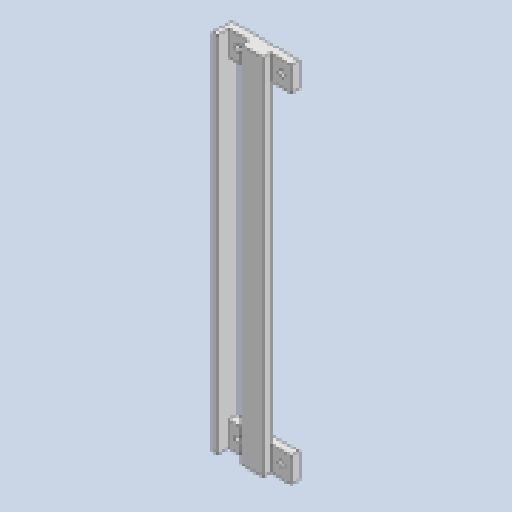
# Autodesk Inventor part: ex_shell_2_wid
Saved by Autodesk Inventor 2023 (Build 270158000, 158)
## iProperties
Created: 2022-10-02
Part Number: ex_shell_2_wid
Material: Generic
Document SubType Name: Modeling
Designer: Shuang Peng
Density: 1 g/cm^3
Appearance: Default
Author: Shuang Peng
Autodesk Inventor part; units mm, degrees
ref_plane "YZ Plane" through (0, 0, 0) normal (1, 0, 0) x (0, 1, 0)
ref_plane "XZ Plane" through (0, 0, 0) normal (0, 1, 0) x (-1, 0, 0)
ref_plane "XY Plane" through (0, 0, 0) normal (0, 0, 1) x (1, 0, 0)
sketch "Sketch1" plane through (0, 0, 0) normal (0, 0, 1) x (1, 0, 0)
  circle A0 centre (17.0691, 112) radius 1.6 projected
  circle A1 centre (3.0691, 112) radius 1.6 projected
  line L0 (20.1383, 116) -> (0, 116) projected
  line L1 (0, 116) -> (0, 108) projected
  line L2 (0, 108) -> (20.1383, 108) projected
  line L3 (20.1383, 116) -> (20.1383, 108) projected
  circle A2 centre (17.0691, 3) radius 1.6 projected
  circle A3 centre (3.0691, 3) radius 1.6 projected
  line L4 (20.1383, -1) -> (0, -1) projected
  line L5 (20.1383, -1) -> (20.1383, 7) projected
  line L6 (0, 7) -> (20.1383, 7) projected
  line L7 (0, -1) -> (0, 7) projected
  circle A4 centre (3.0691, 112) radius 1
  circle A5 centre (17.0691, 112) radius 1
  circle A6 centre (3.0691, 3) radius 1
  circle A7 centre (17.0691, 3) radius 1
  line L8 (10.0691, 116) -> (10.0691, -1)
  point P0 (0, 0)
  dimension "d0" = 2
  dimension "d1" = 2
  dimension "d2" = 2
  dimension "d3" = 2
  constraints: 4 centre point, 4 coincident, 2 end point, 2 midpoint
  measures "d0" diameter of A4
  measures "d1" diameter of A5
  measures "d2" diameter of A6
  measures "d3" diameter of A7
extrude "Extrusion1" add sketch "Sketch1" along normal blind 2 contours A0 | A1 | L3 L2 L8 L0 | L8 L2 L1 L0 | A2 | A3 | L4 L8 L6 L5 | L4 L7 L6 L8
sketch "Sketch2" plane through (0, 0, 2) normal (0, 0, 1) x (1, 0, 0)
  line L0 (20.1383, 7) -> (0, 7) projected
  line L1 (0, 108) -> (20.1383, 108) projected
  line L2 (10.0691, 7) -> (10.0691, 108)
  line L3 (6.5691, -1) -> (13.5691, -1)
  line L4 (13.5691, -1) -> (13.5691, 116)
  line L5 (13.5691, 116) -> (6.5691, 116)
  line L6 (6.5691, 116) -> (6.5691, -1)
  line L7 (6.5691, -1) -> (13.5691, 116) construction
  line L8 (13.5691, -1) -> (6.5691, 116) construction
  point P0 (0, 0)
  point P1 (10.0691, 57.5)
  dimension "d6" = 7
  dimension "d7" = 117
  constraints: 14 end point, 5 midpoint, 2 parallel, 2 perpendicular
  measures "d6" distance of L3.start L3.end
  measures "d7" distance of L4.end L3.end
extrude "Extrusion2" add sketch "Sketch2" along normal mid plane 4
sketch "Sketch3" plane through (0, 0, 0) normal (0, 0, -1) x (-1, 0, 0)
  circle A0 centre (-3.0691, 3) radius 1 projected
  circle A1 centre (-17.0691, 3) radius 1 projected
  circle A2 centre (-17.0691, 112) radius 1 projected
  circle A3 centre (-3.0691, 112) radius 1 projected
  line L0 (0, 108) -> (-6.5691, 108) projected
  line L1 (0, 116) -> (0, 108) projected
  line L2 (-20.1383, 116) -> (0, 116) projected
  line L3 (-20.1383, 108) -> (-20.1383, 116) projected
  line L4 (-13.5691, 108) -> (-20.1383, 108) projected
  line L5 (-13.5691, 108) -> (-13.5691, 7) projected
  line L6 (-20.1383, 7) -> (-13.5691, 7) projected
  line L7 (-20.1383, -1) -> (-20.1383, 7) projected
  line L8 (0, -1) -> (-20.1383, -1) projected
  line L9 (0, 7) -> (0, -1) projected
  line L10 (-6.5691, 7) -> (0, 7) projected
  line L11 (-6.5691, 7) -> (-6.5691, 108) projected
  line L12 (-13.5691, 108) -> (-20.1383, 108) projected
  line L13 (-13.5691, 108) -> (-6.5691, 108)
  line L14 (-13.5691, 7) -> (-13.5691, -1) projected
  line L15 (-13.5691, 7) -> (-6.5691, 7)
  point P0 (0, 0)
  constraints: 4 end point, 1 collinear, 1 perpendicular
extrude "Extrusion3" cut sketch "Sketch3" against normal blind 2 contours L11 L15 L5 L13
thicken "Thicken1" operation add thickness 1 both sides no extend neighbours no toward (0, 0, 1) faces at (11.2358, 77, 4)
thicken "Thicken2" operation add thickness 0.5 both sides no extend neighbours no toward (0, 0, 1) faces at (14.4025, 3, 2)
thicken "Thicken3" operation add thickness 0.5 both sides no extend neighbours no toward (0, 0, 1) faces at (5.7358, 3, 2)
thicken "Thicken4" operation add thickness 0.5 both sides no extend neighbours no toward (0, 0, 1) faces at (14.4025, 112, 2)
thicken "Thicken5" operation add thickness 0.5 both sides no extend neighbours no toward (0, 0, 1) faces at (5.7358, 112, 2)
sketch "Sketch4" plane through (0, -1, 0) normal (-1, 0, 0) x (0, 0, 1)
  line L0 (0, 8) -> (0, 0) projected
  line L1 (0, 0) -> (2.5, 0) projected
  line L2 (2.5, 8) -> (2.5, 0) projected
  line L3 (0, 8) -> (2.5, 8) projected
  line L4 (0, 117) -> (0, 109) projected
  line L5 (0, 109) -> (2.5, 109) projected
  line L6 (2.5, 117) -> (2.5, 109) projected
  line L7 (0, 117) -> (2.5, 117) projected
  line L8 (0, 0) -> (6, 0)
  line L9 (6, 0) -> (6, 117)
  line L10 (6, 117) -> (0, 117)
  line L11 (0, 117) -> (0, 0)
  point P0 (0, 1)
  dimension "d22" = 6
  dimension "d23" = 117
  constraints: 8 end point, 2 parallel, 1 horizontal, 1 perpendicular
  measures "d22" distance of L10.end L9.end
  measures "d23" distance of L9.end L8.end
extrude "Extrusion4" add sketch "Sketch4" along normal blind 2
ref_plane "Work Plane1" through (6.5691, 57.5, 5) normal (0, -1, 0) x (1, 0, 0)
sketch "Sketch5" plane through (6.5691, 57.5, 5) normal (0, -1, 0) x (1, 0, 0)
  line L0 (-6.5691, -5) -> (7, -3)
  line L1 (7, -3) -> (7, 0)
  line L2 (7, 0) -> (-6.5691, 1)
  line L3 (-6.5691, 1) -> (-8.5691, 1)
  line L4 (-8.5691, 1) -> (-8.5691, -5)
  line L5 (-8.5691, -5) -> (-6.5691, -5)
  constraints: 12 end point, 2 perpendicular, 1 vertical
extrude "Extrusion5" add sketch "Sketch5" along normal mid plane 2
pattern_linear "Rectangular Pattern1" count 2 spacing 30 along (0, 1, 0) count 2 spacing 30 along (0, -1, 0) of "Extrusion5"
body "Solid1"
